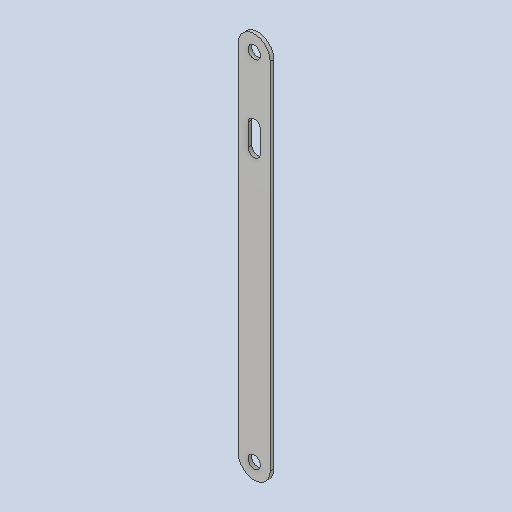
# Autodesk Inventor part: foot_link_lever
Saved by Autodesk Inventor 2022 (Build 260153000, 153)
## iProperties
Category: リンク
Created: 2016-08-23
Part Number: foot_link_lever
Material: GFRP
Document SubType Name: Modeling
Designer: hiro
Density: 1.75 g/cm^3
Appearance: 滑らか - 淡い灰色
Mass: 6.98824 g
Surface Area: 46.6416 cm^2
Volume: 3.99328 cm^3
Author: hiro
Autodesk Inventor part; units mm, degrees
ref_plane "YZ Plane" through (0, 0, 0) normal (1, 0, 0) x (0, 1, 0)
ref_plane "XZ Plane" through (0, 0, 0) normal (0, 1, 0) x (-1, 0, 0)
ref_plane "XY Plane" through (0, 0, 0) normal (0, 0, 1) x (1, 0, 0)
sketch "スケッチ1" plane through (0, 0, 0) normal (0, 0, 1) x (1, 0, 0)
  line L0 (18, 0) -> (18, 200)
  line L1 (0, 200) -> (0, 0)
  line L2 (9, 200) -> (9, 0) construction
  arc A0 (18, 200) -> (0, 200) centre (9, 200) ccw
  arc A1 (0, 0) -> (18, 0) centre (9, 0) ccw
  circle A2 centre (9, 0) radius 3.5
  circle A3 centre (9, 200) radius 3.5
  dimension "d35" = 18
  dimension "d36" = 200
  dimension "d37" = 7
  dimension "d38" = 7
  constraints: 6 end point, 4 centre point, 4 coincident, 4 point on circle, 2 horizontal alignment, 1 parallel
  measures "d35" distance of L0.start L1.end
  measures "d36" distance of L1.start L1.end
  measures "d37" diameter of A2
  measures "d38" diameter of A3
extrude "押し出し1" add sketch "スケッチ1" along normal blind 2
sketch "スケッチ3" plane through (0, 0, 2) normal (0, 0, 1) x (1, 0, 0)
  circle A0 centre (9, 0) radius 3.5 projected
  circle A1 centre (9, 200) radius 3.5 projected
  arc A2 (18, 200) -> (0, 200) centre (9, 200) ccw projected
  line L0 (0, 200) -> (0, 0) projected
  arc A3 (0, 0) -> (18, 0) centre (9, 0) ccw projected
  line L1 (18, 0) -> (18, 200) projected
  circle A4 centre (9, 0) radius 3.5 projected
  line L2 (9, 200) -> (9, 0) construction
  arc A5 (5.5, 152) -> (12.5, 152) centre (9, 152) ccw
  arc A6 (12.5, 164) -> (5.5, 164) centre (9, 164) ccw
  line L3 (5.5, 164) -> (5.5, 152)
  line L4 (12.5, 164) -> (12.5, 152)
  dimension "d41" = 7
  dimension "d42" = 48
  dimension "d43" = 7
  dimension "d44" = 36
  constraints: 6 end point, 4 point on circle, 3 tangent, 2 centre point, 2 point on line, 1 vertical
  measures "d41" diameter of A5
  measures "d42" distance of A5.centre A1.centre
  measures "d43" diameter of A6
  measures "d44" distance of A6.centre A1.centre
extrude "押し出し2" cut sketch "スケッチ3" against normal through all contours L3 A6 L4 A5
